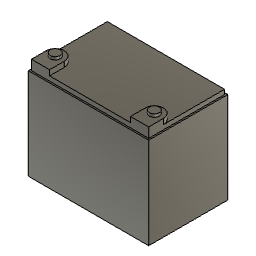
Battery v1 (Autodesk Fusion 360 design; units mm, degrees)
Autodesk Fusion 360 part; units mm, degrees
sketch "Sketch1" plane through (0, 0, 0) normal (0, 0, 1) x (1, 0, 0)
  line L0 (96, -63) -> (-96, -63)
  line L1 (-96, -63) -> (-96, 63)
  line L2 (-96, 63) -> (96, 63)
  line L3 (96, 63) -> (96, -63)
  line L4 (96, -63) -> (-96, 63) construction
  line L5 (-96, -63) -> (96, 63) construction
  dimension "d1" = 192
  dimension "d2" = 126
  constraint horizontal L0
  constraint perpendicular L0 L1
  constraint parallel L0 L2
  constraint parallel L1 L3
  constraint coincident L4 origin
  constraint coincident L5 origin
  measures "d1" distance of L1.end L2.end
  measures "d2" distance of L0.end L1.end
extrude "Extrude1" add sketch "Sketch1" along normal blind 145.75
sketch "Sketch4" plane through (0, 0, 145.75) normal (0, 0, 1) x (-1, 0, 0)
  line L0 (-96, -63) -> (96, -63)
  line L1 (96, -63) -> (96, 63)
  line L2 (96, 63) -> (-96, 63)
  line L3 (-96, 63) -> (-96, -63)
  line L4 (96, -63) -> (-96, -63)
  line L5 (-96, -63) -> (-96, 63)
  line L6 (-96, 63) -> (96, 63)
  line L7 (96, 63) -> (96, -63)
  line L8 (-93.5, 60.5) -> (93.5, 60.5)
  line L9 (93.5, 60.5) -> (93.5, -60.5)
  line L10 (93.5, -60.5) -> (-93.5, -60.5)
  line L11 (-93.5, -60.5) -> (-93.5, 60.5)
  dimension "d12" = 2.5
  constraint horizontal L4
  constraint vertical L5
  constraint horizontal L6
  constraint vertical L7
  constraint coincident L2.end L3.start
  constraint coincident L0.end L1.start
extrude "Extrude4" add sketch "Sketch4" along normal blind 7.25 contours L8 L9 L10 L11
sketch "Sketch5" plane through (0, 0, 153) normal (0, 0, 1) x (-1, 0, 0)
  line L0 (-93.5, -60.5) -> (93.5, -60.5)
  line L1 (93.5, -60.5) -> (93.5, 60.5)
  line L2 (93.5, 60.5) -> (-93.5, 60.5)
  line L3 (-93.5, 60.5) -> (-93.5, -60.5)
  line L4 (93.5, 60.5) -> (64.5, 60.5)
  line L5 (64.5, 60.5) -> (64.5, 37)
  line L6 (93.5, 37) -> (93.5, 60.5)
  line L7 (-93.5, 60.5) -> (-64.5, 60.5)
  line L8 (-64.5, 60.5) -> (-64.5, 37)
  line L9 (-93.5, 37) -> (-93.5, 60.5)
  arc A0 (64.5, 37) -> (93.5, 37) centre (79, 37) ccw
  arc A1 (-93.5, 37) -> (-64.5, 37) centre (-79, 37) ccw
  dimension "d15" = 14.5
  dimension "d16" = 23.5
  constraint horizontal L4
  constraint vertical L5
  constraint vertical L6
  constraint coincident L1.end L2.start
  constraint horizontal L7
  constraint vertical L8
  constraint vertical L9
  constraint coincident L2.end L3.start
  constraint tangent L6 A0
  constraint tangent L5 A0
  constraint tangent L8 A1
  constraint tangent L9 A1
  constraint equal A0 A1
  constraint equal L5 L8
  measures "d15" radius of A0
  measures "d16" distance of L4.end L5.end
extrude "Extrude5" add sketch "Sketch5" along normal blind 8.5 contours L2 L3 L7 L8 L9 A1 | L1 L2 L4 L5 L6 A0
sketch "Sketch6" plane through (0, 0, 161.5) normal (0, 0, 1) x (-1, 0, 0)
  arc A0 (64.5, 37) -> (93.5, 37) centre (79, 37) ccw
  line L0 (93.5, 37) -> (93.5, 60.5)
  line L1 (93.5, 60.5) -> (64.5, 60.5)
  line L2 (64.5, 60.5) -> (64.5, 37)
  circle A1 centre (79, 37) radius 8
  circle A2 centre (-79, 37) radius 8
  arc A3 (-93.5, 37) -> (-64.5, 37) centre (-79, 37) ccw
  dimension "d19" = 16
  constraint concentric A0 A1
  constraint concentric A2 A3
  constraint equal A1 A2
  measures "d19" diameter of A1
extrude "Extrude6" add sketch "Sketch6" along normal blind 4.6 contours A1 | A2
equation "d3 = 153 mm - 7.25 mm"
equation "d16 = 38 mm - 14.5 mm"
